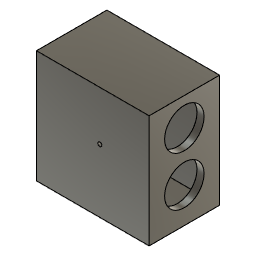
USB CarPower Block v2 (Autodesk Fusion 360 design; units mm, degrees)
Autodesk Fusion 360 part; units mm, degrees
sketch "Sketch1" plane through (0, 0, 0) normal (0, 0, 1) x (1, 0, 0)
  line L0 (-20, 20) -> (60, 20)
  line L1 (60, 20) -> (60, -30)
  line L2 (60, -30) -> (-20, -30)
  line L3 (-20, -30) -> (-20, 20)
  dimension "d1" = 80
  dimension "d2" = 50
  constraint horizontal L0
  constraint vertical L1
  constraint horizontal L2
  constraint vertical L3
  measures "d1" distance of L0.start L0.end
  measures "d2" distance of L0.start L2.end
extrude "Extrude1" add sketch "Sketch1" along normal blind 80
cylinder "CylinderPrimitive1" cut diameter 28 height -100 placed x (0, 0, -1) y (0, 1, 0) z (1, 0, 0) at (60, -5, 25)
cylinder "CylinderPrimitive2" cut diameter 28 height -95 placed x (0, 0, -1) y (0, 1, 0) z (1, 0, 0) at (60, -5, 60)
box "BoxPrimitive1" cut length 73.4567 width 43.5237 height -75 placed x (0, 0, -1) y (0, -1, 0) z (-1, 0, 0) at (-20, 16.7884, 76.3145)
cylinder "CylinderPrimitive3" cut diameter 2.84 height -65 placed x (1, 0, 0) y (0, 0, 1) z (0, -1, 0) at (25, -30, 45)
